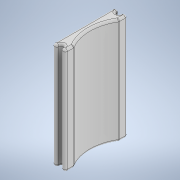
# Autodesk Inventor part: CableCapV1.stl
Saved by Autodesk Inventor 2020 (Build 240168000, 168)
## iProperties
Created: 2020-07-30
Part Number: CableCapV1.stl
Material: Generic
Document SubType Name: Modeling
Designer: maple
Density: 1 g/cm^3
Appearance: Default
Author: maple
Autodesk Inventor part; units mm, degrees
ref_plane "YZ Plane" through (0, 0, 0) normal (1, 0, 0) x (0, 1, 0)
ref_plane "XZ Plane" through (0, 0, 0) normal (0, 1, 0) x (-1, 0, 0)
ref_plane "XY Plane" through (0, 0, 0) normal (0, 0, 1) x (1, 0, 0)
sketch "Sketch1" plane through (0, 0, 0) normal (0, 1, 0) x (-1, 0, 0)
  line L0 (0, 0) -> (0, -25.2476)
  line L1 (0, -25.2476) -> (-2, -25.2476)
  line L2 (-2, -25.2476) -> (-2, -27.2476)
  line L3 (-2, -27.2476) -> (0, -27.2476)
  line L4 (0, -27.2476) -> (0, -25.2476)
  line L5 (-2, -25.2476) -> (4, -25.2476)
  line L6 (4, -25.2476) -> (4, -23.2476)
  line L7 (4, -23.2476) -> (-2, -23.2476)
  line L8 (-2, -23.2476) -> (-2, -25.2476)
  line L9 (4, -25.2476) -> (2, -25.2476)
  line L10 (2, -25.2476) -> (2, -27.2476)
  line L11 (2, -27.2476) -> (4, -27.2476)
  line L12 (4, -27.2476) -> (4, -25.2476)
  line L13 (0, 0) -> (-2, 0)
  line L14 (-2, 0) -> (-2, 2)
  line L15 (-2, 2) -> (0, 2)
  line L16 (0, 2) -> (0, 0)
  line L17 (-2, 0) -> (4, 0)
  line L18 (4, 0) -> (4, -2)
  line L19 (4, -2) -> (-2, -2)
  line L20 (-2, -2) -> (-2, 0)
  line L21 (4, 0) -> (2, 0)
  line L22 (2, 0) -> (2, 2)
  line L23 (2, 2) -> (4, 2)
  line L24 (4, 2) -> (4, 0)
  line L25 (4, -2) -> (4, -23.2476)
  arc A0 (-2, -23.2476) -> (-2, -2) centre (-19.3109, -12.6238) ccw
  dimension "d0" = 25.2476
  dimension "d1" = 2
  dimension "d2" = 2
  dimension "d3" = 6
  dimension "d4" = 2
  dimension "d5" = 2
  dimension "d6" = 2
  dimension "d7" = 2
  dimension "d8" = 2
  dimension "d9" = 6
  dimension "d10" = 2
  dimension "d11" = 2
  dimension "d12" = 2
  constraints: 52 end point, 12 parallel, 6 horizontal, 6 perpendicular, 2 point on circle, 1 centre point, 1 vertical
  measures "d0" distance of L0.start L0.end
  measures "d1" distance of L3.end L2.end
  measures "d2" distance of L2.end L1.end
  measures "d3" distance of L7.end L6.end
  measures "d4" distance of L6.end L5.end
  measures "d5" distance of L11.end L10.end
  measures "d6" distance of L10.end L9.end
  measures "d7" distance of L14.end L15.end
  measures "d8" distance of L13.end L14.end
  measures "d9" distance of L18.end L19.end
  measures "d10" distance of L17.end L18.end
  measures "d11" distance of L22.end L23.end
  measures "d12" distance of L21.end L22.end
extrude "Extrusion1" add sketch "Sketch1" along normal blind 50 contours L17 L18 L19 L0 | L0 L19 L20 L13 | L13 L14 L15 L16 | L19 L25 L7 L0 A0 | L0 A0 L19 | L22 L23 L24 L17 | L0 L7 A0 | L6 L5 L0 L7 | L0 L1 L8 L7 | L12 L11 L10 L5 | L4 L3 L2 L1
fillet "Fillet1" radius 1 14 edges at (-4, 25, -27.2476) (-2, 25, -27.2476) (-2, 25, -25.2476) (0, 25, -25.2476) (0, 25, -27.2476) (2, 25, -27.2476) (2, 25, 2) (0, 25, 2) (0, 25, 0) (-2, 25, 0) (-2, 25, 2) (-4, 25, 2) (2, 25, -2) (2, 25, -23.2476)
fillet "Fillet2" radius 1 38 edges at (1.9642, 0, -23.261) (2, 0, -25.7477) (0, 0, -26.2476) (0.2929, 0, -26.9547) (1, 0, -27.2476) (-2, 0, -26.2476) (-1, 0, -25.2476) (-3.7071, 0, -26.9547) (-3, 0, -27.2476) (-4, 0, -24.2476) (-3, 0, 2) (-2.2929, 0, 1.7071) (-2, 0, 1) (-1, 0, 0) (0, 0, 1) (1.7071, 0, 1.7071) (2, 0, 0.5001) (1.9642, 0, -1.9866) (-1, 0, -12.6238) (-3, 50, 2) (-2.2929, 50, 1.7071) (-2, 50, 1) (-1, 50, 0) (0, 50, 1) (1.7071, 50, 1.7071) (2, 50, 0.5001) (1.9642, 50, -1.9866) (-1, 50, -12.6238) (1.9642, 50, -23.261) (2, 50, -25.7477) (0, 50, -26.2476) (0.2929, 50, -26.9547) (1, 50, -27.2476) (-2, 50, -26.2476) (-1, 50, -25.2476) (-3.7071, 50, -26.9547) (-3, 50, -27.2476) (-4, 50, -24.2476)
body "Solid1"
